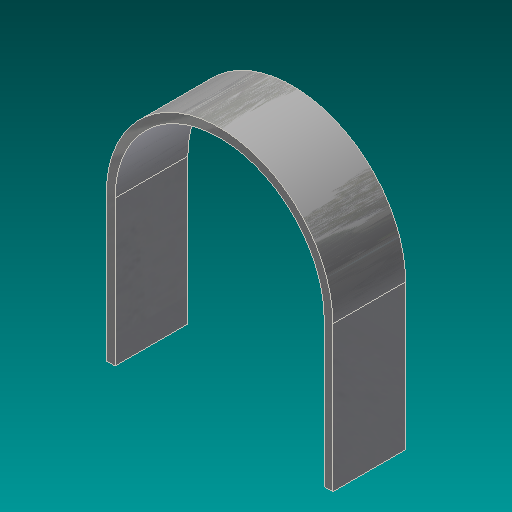
# Autodesk Inventor part: A1-18002-100-50 Tube cradle - 2.875in
Saved by Autodesk Inventor 2017 (Build 210142000, 142)
## iProperties
Created: 2018-06-12
Part Number: A1-18002-100-50 Tube cradle - 2.875in
Material: Steel, Mild
Document SubType Name: Sheet Metal
Designer: Graeme_Van_Dongen
Density: 7.85 g/cm^3
Flat Pattern Width: 2.54 cm
Flat Pattern Length: 22.0521 cm
Flat Pattern Area: 56.0122 cm^2
Sheet Metal Rule: Default
Sheet Metal Width: 1.000 in
Sheet Metal Length: 8.682 in
Sheet Metal Area: 8.682 in^2
Appearance: Steel
Mass: 134.369 g
Surface Area: 127.343 cm^2
Volume: 17.117 cm^3
Author: Graeme_Van_Dongen
Autodesk Inventor part; units mm, degrees
ref_plane "YZ Plane" through (0, 0, 0) normal (1, 0, 0) x (0, 1, 0)
ref_plane "XZ Plane" through (0, 0, 0) normal (0, 1, 0) x (-1, 0, 0)
ref_plane "XY Plane" through (0, 0, 0) normal (0, 0, 1) x (1, 0, 0)
sketch "Sketch1" plane through (0, 0, 0) normal (0, 0, 1) x (1, 0, 0)
  arc A0 (36.5125, 0) -> (-36.5125, 0) centre (0, 0) ccw
  line L0 (36.5125, 0) -> (36.5125, -50.8)
  line L1 (36.5125, -50.8) -> (39.5605, -50.8)
  line L2 (39.5605, -50.8) -> (39.5605, 0)
  arc A1 (39.5605, 0) -> (-39.5605, 0) centre (0, 0) ccw
  line L3 (-39.5605, 0) -> (-39.5605, -50.8)
  line L4 (-39.5605, -50.8) -> (-36.5125, -50.8)
  line L5 (-36.5125, -50.8) -> (-36.5125, 0)
  dimension "d0" = 73.025
  dimension "d1" = 3.048
  dimension "d2" = 50.8
  constraints: 12 end point, 4 perpendicular, 4 point on circle, 4 tangent, 2 centre point, 2 vertical, 1 coincident, 1 concentric, 1 parallel
  measures "d0" diameter of A0
  measures "d1" distance of L0.end L1.end
  measures "d2" distance of L1.end L2.end
extrude "Extrusion1" add sketch "Sketch1" along normal blind 25.4
equation "\"d1\" = Thickness"
equation "\"BendRadius\" = Thickness"
equation "\"BendReliefWidth\" = Thickness"
equation "\"BendReliefDepth\" = 0.5 * Thickness"
equation "\"CornerReliefSize\" = 4 * Thickness"
equation "\"MinimumRemnant\" = 2 * Thickness"
equation "\"TransitionRadius\" = BendRadius"
equation "\"JacobiRadiusSize\" = Thickness"
equation "\"GapSize\" = Thickness"
equation "\"Thickness\" = 3.048"
body "Solid1"
